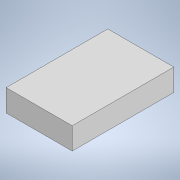
# Autodesk Inventor part: Electronics place holder
Saved by Autodesk Inventor 2020 (Build 240168000, 168)
## iProperties
Created: 2020-04-09
Part Number: Electronics place holder
Material: Generic
Document SubType Name: Modeling
Designer: angusaitken
Density: 1 g/cm^3
Appearance: Default
Author: angusaitken
Autodesk Inventor part; units mm, degrees
ref_plane "YZ Plane" through (0, 0, 0) normal (1, 0, 0) x (0, 1, 0)
ref_plane "XZ Plane" through (0, 0, 0) normal (0, 1, 0) x (-1, 0, 0)
ref_plane "XY Plane" through (0, 0, 0) normal (0, 0, 1) x (1, 0, 0)
sketch "Sketch1" plane through (0, 0, 0) normal (0, 1, 0) x (-1, 0, 0)
  line L0 (0, 0) -> (130, 0)
  line L1 (130, 0) -> (130, -200)
  line L2 (130, -200) -> (0, -200)
  line L3 (0, -200) -> (0, 0)
  dimension "d0" = 130
  dimension "d1" = 200
  constraints: 8 end point, 2 parallel, 1 horizontal, 1 perpendicular
  measures "d0" distance of L1.end L2.end
  measures "d1" distance of L0.end L1.end
extrude "Extrusion1" add sketch "Sketch1" along normal blind 25.4
sketch "Sketch2" plane through (0, 0, 0) normal (0, -1, 0) x (1, 0, 0)
  line L0 (0, -200) -> (-130, -200) projected
  line L1 (0, 0) -> (0, -200) projected
  line L2 (-102.952, -44.8611) -> (-27.048, -44.8611)
  line L3 (-27.048, -44.8611) -> (-27.048, -155.1389)
  line L4 (-27.048, -155.1389) -> (-102.952, -155.1389)
  line L5 (-102.952, -155.1389) -> (-102.952, -44.8611)
  line L6 (-102.952, -44.8611) -> (-27.048, -155.1389) construction
  line L7 (-27.048, -44.8611) -> (-102.952, -155.1389) construction
  line L8 (-130, -200) -> (-130, 0) projected
  line L9 (-130, 0) -> (0, 0) projected
  point P0 (-65, -100)
  constraints: 12 end point, 2 midpoint, 2 parallel, 1 horizontal, 1 perpendicular
extrude "Extrusion2" add sketch "Sketch2" along normal blind 17.78
body "Solid1"
